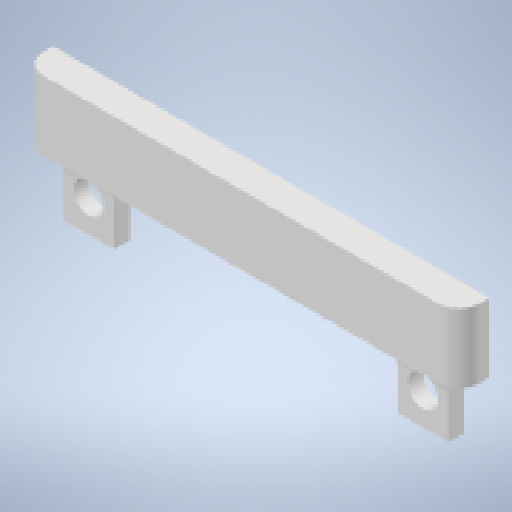
# Autodesk Inventor part: wire_fixs
Saved by Autodesk Inventor 2023 (Build 270158000, 158)
## iProperties
Created: 2026-04-20
Part Number: wire_fixs
Material: Типовые
Document SubType Name: Modeling
Designer: garin
Density: 1 g/cm^3
Appearance: По умолчанию
Author: garin
Autodesk Inventor part; units mm, degrees
ref_plane "YZ Plane" through (0, 0, 0) normal (1, 0, 0) x (0, 1, 0)
ref_plane "XZ Plane" through (0, 0, 0) normal (0, 1, 0) x (-1, 0, 0)
ref_plane "XY Plane" through (0, 0, 0) normal (0, 0, 1) x (1, 0, 0)
sketch "Эскиз1" plane through (0, 0, 0) normal (0, 0, 1) x (1, 0, 0)
  line L0 (0, 0) -> (21.45, 0) construction
  line L1 (21.45, 0) -> (21.45, 46.7) construction
  line L2 (21.45, 46.7) -> (0, 46.7) construction
  line L3 (0, 46.7) -> (0, 0) construction
  line L4 (21.45, 46.7) -> (16.45, 46.7) construction
  line L5 (16.45, 46.7) -> (16.45, 43.8) construction
  line L6 (16.45, 43.8) -> (21.45, 43.8) construction
  line L7 (21.45, 43.8) -> (21.45, 46.7) construction
  circle A0 centre (16.45, 43.8) radius 1.5
  circle A1 centre (-16.45, 43.8) radius 1.5
  line L8 (21.45, 46.7) -> (-21.45, 46.7)
  line L9 (-21.45, 46.7) -> (-21.45, 53.5)
  line L10 (-21.45, 53.5) -> (21.45, 53.5)
  line L11 (21.45, 53.5) -> (21.45, 46.7)
  line L12 (21.45, 46.7) -> (18.95, 46.7)
  line L13 (18.95, 46.7) -> (18.95, 40.7)
  line L14 (18.95, 40.7) -> (13.95, 40.7)
  line L15 (13.95, 40.7) -> (13.95, 46.7)
  line L16 (-16.45, 46.7) -> (-16.45, 43.8) construction
  line L17 (-16.45, 43.8) -> (-21.45, 43.8) construction
  line L18 (-18.95, 46.7) -> (-18.95, 40.7)
  line L19 (-18.95, 40.7) -> (-13.95, 40.7)
  line L20 (-13.95, 40.7) -> (-13.95, 46.7)
  circle A2 centre (-16.45, 43.8) radius 1.5
  dimension "d0" = 21.45
  dimension "d1" = 46.7
  dimension "d2" = 5
  dimension "d3" = 2.9
  dimension "d4" = 3
  dimension "d5" = 42.9
  dimension "d6" = 6.8
  dimension "d7" = 2.5
  dimension "d8" = 6
  dimension "d9" = 5
  constraints: 42 end point, 10 symmetric about line, 6 parallel, 4 horizontal, 4 perpendicular, 3 centre point, 2 coincident, 2 point on line, 1 vertical, 2 other
  measures "d0" distance of L2.end L1.end
  measures "d1" distance of L1.end L0.end
  measures "d2" distance of L6.end L5.end
  measures "d3" distance of L5.end L4.end
  measures "d4" diameter of A0
  measures "d5" distance of L9.end L10.end
  measures "d6" distance of L8.end L9.end
  measures "d7" distance of L1.end L12.end
  measures "d8" distance of L12.end L13.end
  measures "d9" distance of L13.end L14.end
extrude "Выдавливание1" add sketch "Эскиз1" along normal blind 1.5 contours L13 L14 L15 L8 | L20 L19 L18 L8
extrude "Выдавливание2" add sketch "Эскиз1" along normal blind 3 contours L8 L9 L10 L11
fillet "Сопряжение1" radius 2 4 edges at (-21.45, 50.1, 3) (-16.45, 46.7, 1.5) (21.45, 50.1, 3) (16.45, 46.7, 1.5)
